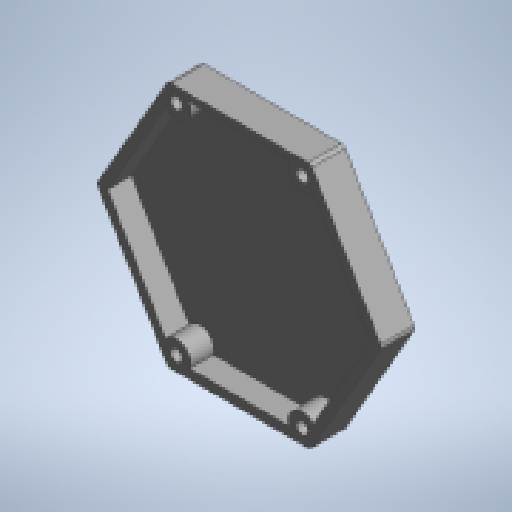
# Autodesk Inventor part: ArmPowerBoardLid2
Saved by Autodesk Inventor 2023 (Build 270158000, 158)
## iProperties
Created: 2023-11-26
Part Number: ArmPowerBoardLid2
Material: Generic
Document SubType Name: Modeling
Designer: LattePanda
Density: 1 g/cm^3
Appearance: Default
Author: LattePanda
Autodesk Inventor part; units mm, degrees
ref_plane "YZ Plane" through (0, 0, 0) normal (1, 0, 0) x (0, 1, 0)
ref_plane "XZ Plane" through (0, 0, 0) normal (0, 1, 0) x (-1, 0, 0)
ref_plane "XY Plane" through (0, 0, 0) normal (0, 0, 1) x (1, 0, 0)
sketch "Sketch1" plane through (0, 0, 0) normal (0, 0, 1) x (1, 0, 0)
  circle A0 centre (27.6906, -3) radius 1 construction
  line L0 (42.1132, -25.9806) -> (29.9708, -4.9495)
  line L1 (29.9708, -47.012) -> (42.1132, -25.9806)
  arc A1 (29.9708, -47.012) -> (24.8622, -49.9615) centre (27.6906, -48.9615) ccw
  line L2 (3.9831, -49.9615) -> (24.8622, -49.9615)
  arc A2 (3.9831, -49.9615) -> (-1.1256, -47.0121) centre (1.1547, -48.9615) ccw
  line L3 (-13.268, -25.9808) -> (-1.1256, -47.0121)
  line L4 (-1.1255, -4.9495) -> (-13.268, -25.9808)
  arc A3 (-1.1255, -4.9495) -> (3.7528, -1.5) centre (1.1547, -3) ccw
  line L5 (25.0925, -1.5) -> (3.7528, -1.5)
  arc A4 (25.0925, -1.5) -> (29.9708, -4.9495) centre (27.6906, -3) ccw
  line L6 (44.1339, -26.4806) -> (29.7113, -51.4615)
  arc A5 (44.1339, -26.4806) -> (44.1339, -25.4806) centre (43.2679, -25.9806) ccw
  line L7 (29.7113, -0.5) -> (44.1339, -25.4806)
  arc A6 (29.7113, -0.5) -> (28.8453, 0) centre (28.8453, -1) ccw
  line L8 (0, 0) -> (28.8453, 0)
  arc A7 (0, 0) -> (-0.866, -0.5) centre (0, -1) ccw
  line L9 (-15.2887, -25.4808) -> (-0.866, -0.5)
  arc A8 (-15.2887, -25.4808) -> (-15.2887, -26.4808) centre (-14.4227, -25.9808) ccw
  line L10 (-0.8661, -51.4615) -> (-15.2887, -26.4808)
  arc A9 (-0.8661, -51.4615) -> (-0.0001, -51.9615) centre (-0.0001, -50.9615) ccw
  line L11 (28.8452, -51.9615) -> (-0.0001, -51.9615)
  arc A10 (28.8452, -51.9615) -> (29.7113, -51.4615) centre (28.8452, -50.9615) ccw
  circle A11 centre (1.1547, -48.9615) radius 1 construction
  circle A12 centre (1.1547, -3) radius 1 construction
  line L12 (28.5507, -49.4717) -> (28.5625, -49.4513)
  arc A13 (27.6982, -49.9615) -> (28.5507, -49.4717) centre (27.6906, -48.9615) ccw construction
  line L13 (27.683, -49.9615) -> (27.6982, -49.9615)
  arc A14 (28.5625, -49.4513) -> (27.683, -49.9615) centre (27.6906, -48.9615) ccw construction
  circle A15 centre (1.1547, -3) radius 1.25
  circle A16 centre (27.6906, -3) radius 1.25
  circle A17 centre (1.1547, -48.9615) radius 1.25
  circle A18 centre (27.6906, -48.9615) radius 1.25
  point P0 (14.4226, -25.9808)
  dimension "d4" = 2.5
  dimension "d5" = 2.5
  dimension "d6" = 2.5
  dimension "d7" = 2.5
  constraints: 28 end point, 24 point on circle, 19 centre point, 4 coincident
  measures "d4" diameter of A15
  measures "d5" diameter of A16
  measures "d6" diameter of A17
  measures "d7" diameter of A18
extrude "Extrusion1" add sketch "Sketch1" along normal blind 5
extrude "Extrusion2" add sketch "Sketch1" against normal blind 2 contours L1 A1 L2 A2 L3 L4 A3 L5 A4 L0 | L6 A10 L11 A9 L10 A8 L9 A7 L8 A6 L7 A5 | A15 | A16 | A17 | A18
body "Solid1"
